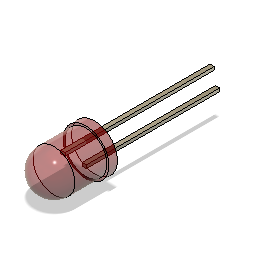
LED 3mm (Red) (Autodesk Fusion 360 design; units mm, degrees)
Autodesk Fusion 360 part; units mm, degrees
sketch "Sketch1" plane through (0, 0, 0) normal (0, 1, 0) x (1, 0, 0)
  circle A0 centre (0, 0) radius 2.7305
  circle A1 centre (0, 0) radius 2.4892
  dimension "d1" = 5.461
  dimension "d2" = 4.9784
  constraint coincident A0.centre A1.centre
  constraint concentric A0 A1
  measures "d1" diameter of A0
  measures "d2" diameter of A1
extrude "Extrude1" add sketch "Sketch1" along normal blind 1.016 contours A0 | A1 makes body 1
extrude "Extrude2" add sketch "Sketch1" against normal blind 3.81 contours A1 bodies 1
ref_plane "WorkPlane1" through (2.4892, -2.871, 0) normal (1, 0, 0) x (0, 0, -1)
ref_plane "WorkPlane2" through (0, -2.871, 0) normal (1, 0, 0) x (0, 0, -1)
sketch "Sketch3" plane through (0, -2.871, 0) normal (1, 0, 0) x (0, 0, -1)
  line L0 (-2.4892, -0.939) -> (2.4892, -0.939)
  line L1 (0, -0.939) -> (0, -3.4282)
  arc A0 (0, -3.4282) -> (2.4892, -0.939) centre (0, -0.939) ccw
  dimension "d9" = 2.4892
  constraint midpoint L0 L1.start
  constraint perpendicular L0 L1
  constraint coincident L0.end A0.end
  measures "d9" distance of L1.start L1.end
revolve "Revolve1" add sketch "Sketch3" angle 360 about axis through (0, 0, 0) along (0, 1, 0) bodies 1
sketch "Sketch4" plane through (0, 1.016, 0) normal (0, 1, 0) x (-1, 0, 0)
  circle A0 centre (0, 0) radius 2.7305
  line L0 (1.016, 0.1905) -> (1.524, 0.1905)
  line L1 (1.524, 0.1905) -> (1.524, -0.1905)
  line L2 (1.524, -0.1905) -> (1.016, -0.1905)
  line L3 (1.016, -0.1905) -> (1.016, 0.1905)
  line L4 (1.016, 0.1905) -> (1.524, -0.1905) construction
  line L5 (1.524, 0.1905) -> (1.016, -0.1905) construction
  line L6 (-1.524, 0.1905) -> (-1.016, 0.1905)
  line L7 (-1.016, 0.1905) -> (-1.016, -0.1905)
  line L8 (-1.016, -0.1905) -> (-1.524, -0.1905)
  line L9 (-1.524, -0.1905) -> (-1.524, 0.1905)
  line L10 (-1.524, 0.1905) -> (-1.016, -0.1905) construction
  line L11 (-1.016, 0.1905) -> (-1.524, -0.1905) construction
  point P0 (1.27, 0)
  point P1 (-1.27, 0)
  point P2 (1.27, 0)
  point P3 (-1.27, 0)
  dimension "d11" = 1.27
  dimension "d12" = 1.27
  dimension "d13" = 0.508
  dimension "d14" = 0.381
  dimension "d15" = 0.508
  dimension "d16" = 0.381
  constraint perpendicular L0 L1
  constraint parallel L0 L2
  constraint parallel L1 L3
  constraint horizontal L0
  constraint coincident L4 P2
  constraint coincident L5 P2
  constraint coincident P0 P2
  constraint perpendicular L6 L7
  constraint parallel L6 L8
  constraint parallel L7 L9
  constraint horizontal L6
  constraint coincident L10 P3
  constraint coincident L11 P3
  constraint coincident P1 P3
  measures "d11" distance of A0.centre P2
  measures "d12" distance of A0.centre P1
  measures "d13" distance of L1.end L2.end
  measures "d14" distance of L0.end L1.end
  measures "d15" distance of L7.end L8.end
  measures "d16" distance of L6.end L7.end
extrude "Extrude3" add sketch "Sketch4" along normal blind 17.78 contours L0 L1 L2 L3 bodies 1
extrude "Extrude4" add sketch "Sketch4" along normal blind 15.875 contours L6 L7 L8 L9 bodies 1
split "Split1" by plane through (0, 1.016, 0) normal (0, 1, 0) bodies 1 makes body 2 at (-1.3547, 6.9427, -0.1905) makes body 3 at (1.1853, 11.5993, 0.1905)
move_body "Move1" bodies 1 3 2 to x (1, 0, 0) y (0, 0, -1) z (0, 1, 0) at (0, -3.5687, -9.0297)
move_body "Move2" bodies 1 3 2 to x (1, 0, 0) y (0, 1, 0) z (0, 0, 1) at (0, 6.3104, 10.042)
move_body "Move3" bodies 2 3 to x (1, 0, 0) y (0, 1, 0) z (0, 0, 1) at (0, 0, 2.4836)
equation "d8 = ( -0.196 / 2 ) * 1 in"
equation "d9 = ( 0.196 / 2 ) * 1 in"
named bodies: "Body", "terminal pos", "terminal neg"
